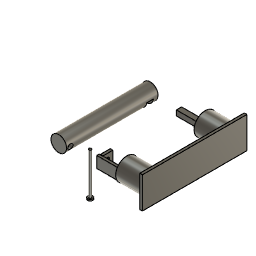
Ninja star holder v4 (Autodesk Fusion 360 design; units mm, degrees)
Autodesk Fusion 360 part; units mm, degrees
sketch "Sketch3" plane through (0, 0, 0) normal (1, 0, 0) x (0, 1, 0) in component "Main"
  line L0 (20, -6) -> (-20, -6)
  line L1 (-20, -6) -> (-20, 6)
  line L2 (-20, 6) -> (20, 6)
  line L3 (20, 6) -> (20, -6)
  line L4 (20, -6) -> (-20, 6) construction
  line L5 (-20, -6) -> (20, 6) construction
  dimension "d3" = 40
  dimension "d4" = 12
  constraint horizontal L0
  constraint perpendicular L0 L1
  constraint parallel L0 L2
  constraint parallel L1 L3
  constraint coincident L4 origin
  constraint coincident L5 origin
  measures "d3" distance of L1.end L2.end
  measures "d4" distance of L0.end L1.end
extrude "Extrude1" add sketch "Sketch3" along normal blind 1 makes body 1 in component "Main"
sketch "Sketch5" plane through (0, 0, 0) normal (-1, 0, 0) x (0, -1, 0) in component "Main"
  line L0 (20, 6) -> (-20, 6)
  line L1 (-20, 6) -> (-20, -6)
  line L2 (-20, -6) -> (20, -6)
  line L3 (20, -6) -> (20, 6)
  circle A0 centre (15, 0) radius 4.25
  circle A1 centre (-15, 0) radius 4.25
  dimension "d8" = 8.5
  dimension "d9" = 8.5
  measures "d8" diameter of A0
  measures "d9" diameter of A1
extrude "Extrude2" add sketch "Sketch5" along normal blind 15 contours A0 bodies 1 in component "Main"
extrude "Extrude3" add sketch "Sketch5" along normal blind 15 contours A1 bodies 1 in component "Main"
sketch "Sketch8" plane through (-15, 0, 0) normal (-1, 0, 0) x (0, -1, 0) in component "Main"
  circle A0 centre (15, 0) radius 4.25
  circle A1 centre (15, 0) radius 4.25
  constraint concentric A0 A1
extrude "Extrude4" cut sketch "Sketch8" against normal blind 5 bodies 1 in component "Main"
sketch "Sketch9" plane through (-10, 0, 0) normal (-1, 0, 0) x (0, -1, 0) in component "Main"
  circle A0 centre (15, 0) radius 4.25
  line L0 (18.5, -2.15) -> (17.5, -2.15)
  line L1 (17.5, -2.15) -> (17.5, 2.15)
  line L2 (17.5, 2.15) -> (18.5, 2.15)
  line L3 (18.5, 2.15) -> (18.5, -2.15)
  line L4 (18.5, -2.15) -> (17.5, 2.15) construction
  line L5 (17.5, -2.15) -> (18.5, 2.15) construction
  point P0 (18, 0)
  dimension "d16" = 1
  dimension "d17" = 4.3
  constraint horizontal L0
  constraint perpendicular L0 L1
  constraint parallel L0 L2
  constraint parallel L1 L3
  constraint coincident L4 P0
  constraint coincident L5 P0
  measures "d16" distance of L1.end L2.end
  measures "d17" distance of L0.end L1.end
extrude "Extrude5" add sketch "Sketch9" along normal blind 8 contours L0 L1 L2 L3 bodies 1 in component "Main"
sketch "Sketch10" plane through (0, -17.5, 0) normal (0, 1, 0) x (-1, 0, 0) in component "Main"
  line L0 (10, 2.15) -> (10, -2.15)
  line L1 (10, -2.15) -> (18, -2.15)
  line L2 (18, -2.15) -> (18, 2.15)
  line L3 (18, 2.15) -> (10, 2.15)
  line L4 (17.8, -2) -> (16.8, -2)
  line L5 (16.8, -2) -> (16.8, 2)
  line L6 (16.8, 2) -> (17.8, 2)
  line L7 (17.8, 2) -> (17.8, -2)
  line L8 (17.8, -2) -> (16.8, 2) construction
  line L9 (16.8, -2) -> (17.8, 2) construction
  point P0 (17.3, 0)
  dimension "d20" = 1
  dimension "d21" = 4
  constraint horizontal L4
  constraint perpendicular L4 L5
  constraint parallel L4 L6
  constraint parallel L5 L7
  constraint coincident L8 P0
  constraint coincident L9 P0
  measures "d20" distance of L5.end L6.end
  measures "d21" distance of L4.end L5.end
extrude "Extrude6" add sketch "Sketch10" along normal blind 4 contours L4 L5 L6 L7 bodies 1 in component "Main"
sketch "Sketch11" plane through (-17.8, 0, 0) normal (-1, 0, 0) x (0, -1, 0) in component "Main"
  line L0 (17.5, -2) -> (17.5, 2)
  line L1 (17.5, 2) -> (13.5, 2)
  line L2 (13.5, 2) -> (13.5, -2)
  line L3 (13.5, -2) -> (17.5, -2)
  circle A0 centre (15.5, 0) radius 1.3
  dimension "d24" = 2.6
  measures "d24" diameter of A0
extrude "Extrude7" cut sketch "Sketch11" against normal blind 0.5 contours A0 bodies 1 in component "Main"
sketch "Sketch12" plane through (-17.3, 0, 0) normal (-1, 0, 0) x (0, -1, 0) in component "Main"
  circle A0 centre (15.5, 0) radius 1.3
  circle A1 centre (15.5, 0) radius 0.65
  dimension "d27" = 1.3
  constraint concentric A0 A1
  measures "d27" diameter of A1
extrude "Extrude8" cut sketch "Sketch12" against normal blind 1.5 contours A1 bodies 1 in component "Main"
extrude "Extrude9" cut 1 faces at (-15, 13.331, 0.9636) along direction (1, 0, 0) blind 5 on bodies 1 bodies 1 in component "Main"
sketch "Sketch13" plane through (-10, 0, 0) normal (-1, 0, 0) x (0, -1, 0) in component "Main"
  circle A0 centre (-15, 0) radius 4.25
  line L0 (-14, -2) -> (-16, -2)
  line L1 (-16, -2) -> (-16, 2)
  line L2 (-16, 2) -> (-14, 2)
  line L3 (-14, 2) -> (-14, -2)
  line L4 (-14, -2) -> (-16, 2) construction
  line L5 (-16, -2) -> (-14, 2) construction
  point P0 (-15, 0)
  dimension "d32" = 2
  constraint horizontal L0
  constraint perpendicular L0 L1
  constraint parallel L0 L2
  constraint parallel L1 L3
  constraint coincident L4 P0
  constraint coincident L5 P0
  constraint coincident P0 A0.centre
  measures "d32" distance of L1.end L2.end
extrude "Extrude10" add sketch "Sketch13" along normal blind 10 contours L0 L1 L2 L3 bodies 1 in component "Main"
move_body "Move1" bodies 1 to x (1, 0, 0) y (0, 1, 0) z (0, 0, 1) at (45, 0, 0) in component "Main"
sketch "Sketch1" plane through (0, 0, 0) normal (0, 0, 1) x (1, 0, 0) in component "Peg"
  circle A0 centre (0, 0) radius 1
  dimension "d35" = 2
  constraint coincident A0.centre origin
  measures "d35" diameter of A0
extrude "Extrude1'" add sketch "Sketch1" along normal blind 0.5 separate body makes body 2 in component "Peg"
sketch "Sketch2" plane through (0, 0, 0.5) normal (0, 0, 1) x (-1, 0, 0) in component "Peg"
  circle A0 centre (0, 0) radius 1
  circle A1 centre (0, 0) radius 0.5
  dimension "d38" = 1
  constraint concentric A0 A1
  measures "d38" diameter of A1
extrude "Extrude2'" add sketch "Sketch2" along normal blind 16 contours A1 bodies 2 in component "Peg"
move_body "Move2" bodies 2 to x (1, 0, 0) y (0, 1, 0) z (0, 0, 1) at (38, -32, 0) in component "Peg"
sketch "Sketch2 (2)" plane through (0, 0, 0) normal (0, 1, 0) x (1, 0, 0) in component "Acton bar"
  circle A0 centre (4, -5) radius 3
  dimension "d41" = 6
  measures "d41" diameter of A0
extrude "Extrude1''" add sketch "Sketch2 (2)" along normal blind 35 separate body makes body 3 in component "Acton bar"
move_body "Move1'" bodies 3 to x (1, 0, 0) y (0, 1, 0) z (0, 0, 1) at (0, -18, 0) in component "Acton bar"
move_face "MoveFace1" to x (1, 0, 0) y (0, 1, 0) z (0, 0, 1) at (24.9633, 0, 1.3549) 1 faces at (6.9851, 5.3333, 5.2987) on bodies 3 in component "Acton bar"
move_body "Move2'" bodies 3 to x (1, 0, 0) y (0, 1, 0) z (0, 0, 1) at (2, 1, 0) in component "Acton bar"
sketch "Sketch3 (2)" plane through (0, 0, 0) normal (1, 0, 0) x (0, 1, 0) in component "Acton bar"
  circle A0 centre (-15.5, 6) radius 1
  dimension "d44" = 2
  measures "d44" diameter of A0
extrude "Extrude2''" cut sketch "Sketch3 (2)" along normal blind 35 bodies 3 in component "Acton bar"
sketch "Sketch4" plane through (0, 0, 0) normal (0, 0, 1) x (1, 0, 0) in component "Acton bar"
  line L0 (35, 13.7403) -> (20.6801, 13.7403)
  line L1 (20.6801, 13.7403) -> (20.6801, 16.2815)
  line L2 (20.6801, 16.2815) -> (35, 16.2815)
  line L3 (35, 16.2815) -> (35, 13.7403)
  constraint horizontal L0
  constraint vertical L1
  constraint horizontal L2
  constraint vertical L3
extrude "Extrude11" cut sketch "Sketch4" along normal blind 6 bodies 1 in component "Main"
extrude "Extrude3'" cut sketch "Sketch4" along normal blind 6 bodies 3 in component "Acton bar"
move_body "Move4" bodies 3 to x (1, 0, 0) y (0, 1, 0) z (0, 0, 1) at (-19.984, 0, -9.0355) in component "Acton bar"
sketch "Sketch14" plane through (35, 0, 0) normal (-1, 0, 0) x (0, -1, 0) in component "Main"
  line L0 (18.5, 2.15) -> (18.5, -2.15)
  line L1 (18.5, -2.15) -> (17.5, -2.15)
  line L2 (17.5, -2.15) -> (17.5, 2.15)
  line L3 (17.5, 2.15) -> (18.5, 2.15)
  circle A0 centre (15, 0) radius 4.25
  circle A1 centre (15.5, 0) radius 0.6403
extrude "Extrude12" cut sketch "Sketch14" against normal blind 10 contours A1 bodies 1 in component "Main"
component "Main" placed x (1, 0, 0) y (0, 1, 0) z (0, 0, 1) at (0, 0, 0)
component "Peg" placed x (1, 0, 0) y (0, 1, 0) z (0, 0, 1) at (0, 0, 0)
component "Acton bar" placed x (1, 0, 0) y (0, 1, 0) z (0, 0, 1) at (0, 0, 0)
